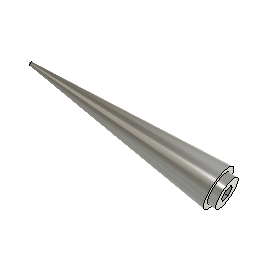
tip (Autodesk Fusion 360 design; units mm, degrees)
Autodesk Fusion 360 part; units mm, degrees
sketch "base" plane through (0, 0, 0) normal (0, 1, 0) x (1, 0, 0)
  circle A0 centre (0, 0) radius 12.75
  circle A1 centre (0, 0) radius 9.5
  line L0 (4.6976, 0.5881) -> (1.8395, 4.3623)
  line L1 (1.8395, 4.3623) -> (-2.8581, 3.7742)
  line L2 (-2.8581, 3.7742) -> (-4.6976, -0.5881)
  line L3 (-4.6976, -0.5881) -> (-1.8395, -4.3623)
  line L4 (-1.8395, -4.3623) -> (2.8581, -3.7742)
  line L5 (2.8581, -3.7742) -> (4.6976, 0.5881)
  dimension "d1" = 25.5
  dimension "d8" = 19
  dimension "d11" = 4.1
  constraint coincident A0.centre A1.centre
  constraint concentric A0 A1
  measures "d1" diameter of A0
  measures "d8" diameter of A1
  measures "d11" distance of A0.centre L5
sketch "side" plane through (0, 0, 0) normal (0, 0, 1) x (1, 0, 0)
  line L0 (0, 0) -> (0, 115)
  line L1 (0, 0) -> (12.75, 0)
  line L2 (0, 115) -> (1, 115)
  line L3 (1, 115) -> (12.75, 0)
  line L4 (0, 108.2663) -> (1.688, 108.2663)
  dimension "d4" = 115
  dimension "d5" = 12.75
  dimension "d19" = 1
  constraint coincident L0.start L1.start
  constraint vertical L0
  constraint perpendicular L0 L1
  constraint perpendicular L0 L2
  constraint coincident L0 L4.start
  constraint coincident L3 L4.end
  constraint perpendicular L0 L4
  measures "d4" distance of L0.start L0.end
  measures "d5" distance of L0.start L1.end
  measures "d19" distance of L0.end L2.end
revolve "cone" add sketch "side" angle 360 about axis through (0, 0, 0) along (0, 1, 0) makes body 1
extrude "tip_insert" cut sketch "base" along normal blind 5 contours A1 | L0 L1 L2 L3 L4 L5 bodies 1
extrude "shoulder" add sketch "base" along normal blind 10 and the other way blind 5 separate body contours A1 | L0 L1 L2 L3 L4 L5 makes body 2
extrude "Extrude2" cut sketch "base" along normal blind 25 from surface at -5 contours L0 L1 L2 L3 L4 L5 bodies 2
fillet "Fillet1" radius 1 1 edges at (-0.9323, 115, -0.3616) on bodies 1
combine "Combine1" operation add target body 1 tool bodies 2
equation "d1 = base_diam"
equation "base_diam = 25.5 mm"
equation "height = 115 mm"
equation "d4 = height"
equation "d5 = base_diam / 2"
equation "inside_diam = 19 mm"
equation "d8 = inside_diam"
named bodies: "tip", "shoulder"
